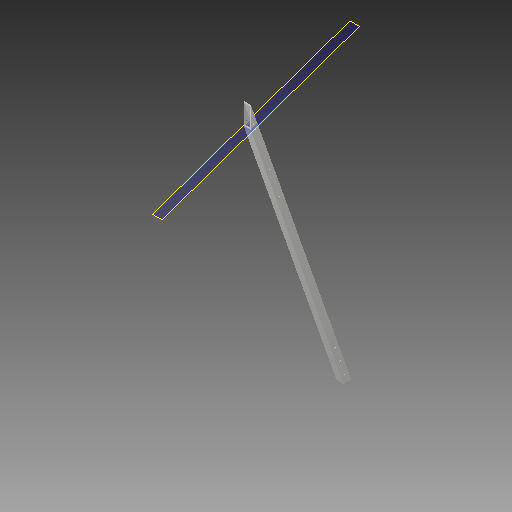
# Autodesk Inventor part: Elevator Support
Saved by Autodesk Inventor 2019.4 (Build 234330000, 330)
## iProperties
Created: 2020-01-09
Part Number: Elevator Support
Material: Aluminum 6061
Document SubType Name: Modeling
Designer: Mark
Mass: 505.998 g
Surface Area: 1886.44 cm^2
Volume: 187.407 cm^3
Density: 2.7 g/cm^3
Appearance: Aluminum - Flat
Author: Mark
Autodesk Inventor part; units mm, degrees
ref_plane "YZ Plane" through (0, 0, 0) normal (1, 0, 0) x (0, 1, 0)
ref_plane "XZ Plane" through (0, 0, 0) normal (0, 1, 0) x (-1, 0, 0)
ref_plane "XY Plane" through (0, 0, 0) normal (0, 0, 1) x (1, 0, 0)
sketch "Sketch2" plane through (0, 0, 0) normal (1, 0, 0) x (0, 1, 0)
  line L0 (0, 0) -> (75.8795, 0)
  line L1 (0, 0) -> (75.8795, 0) construction
  line L2 (-927.1205, -323.5216) -> (-927.1205, -350)
  line L3 (-927.1205, -323.5216) -> (-900.6421, -323.5216) construction
  line L4 (75.8795, 0) -> (-927.1205, -350)
  line L5 (75.8795, 0) -> (-927.1205, -350)
  line L6 (-927.1205, -323.5216) -> (0, 0)
  line L7 (0, 0) -> (75.8795, 0)
  line L8 (-927.1205, -350) -> (-927.1205, -323.5216)
  line L9 (0, 0) -> (-927.1205, -323.5216)
  line L10 (-927.1205, -350) -> (75.8795, 0)
  line L11 (75.8795, 0) -> (0, 0)
  line L12 (-927.1205, -323.5216) -> (-927.1205, -350)
  dimension "d7" = 0
  dimension "d9" = 90
  dimension "d10" = 1003
  dimension "d11" = 350
  dimension "d13" = 25
  constraints: 26 end point, 5 collinear, 4 point on line, 3 horizontal, 2 equal length, 2 parallel, 1 perpendicular, 1 vertical
  measures "d7" distance between parallel lines of L0 L1
  measures "d9" angle of L2 L3
  measures "d10" horizontal distance of L2.start L0.end
  measures "d11" vertical distance of L2.end L0.end
  measures "d13" distance between parallel lines of L4 L6
extrude "Extrusion2" add sketch "Sketch2" along normal blind 25
ref_plane "Work Plane1" through (0, 0, 0) normal (0, -0.9441661, -0.3294697) x (1, 0, 0)
sketch "Sketch3" plane through (0, 0, 0) normal (0, -0.9441661, -0.3294697) x (1, 0, 0)
  line L0 (2, -23) -> (23, -23)
  line L1 (23, -23) -> (23, -2)
  line L2 (23, -2) -> (2, -2)
  line L3 (2, -2) -> (2, -23)
  line L4 (2, -23) -> (23, -2) construction
  line L5 (23, -23) -> (2, -2) construction
  line L6 (25, -25) -> (25, 0) projected
  line L7 (0, 0) -> (25, 0) projected
  point P0 (12.5, -12.5)
  dimension "d17" = 21
  dimension "d18" = 21
  dimension "d19" = 2
  dimension "d20" = 23
  constraints: 12 end point, 2 midpoint, 2 parallel, 1 horizontal, 1 perpendicular
  measures "d17" distance of L2.end L1.end
  measures "d18" distance of L1.end L0.end
  measures "d19" distance between parallel lines of L6 L1
  measures "d20" distance between parallel lines of L7 L0
extrude "Extrusion3" cut sketch "Sketch3" along normal mid plane 2115.25
sketch "Sketch4" plane through (0, 0, 0) normal (-1, 0, 0) x (0, 0, 1)
  circle A0 centre (-65.5822, -150) radius 2.75
  circle A1 centre (-100.1765, -249.1374) radius 2.75
  line L0 (-323.5216, -927.1205) -> (0, 0) projected
  line L1 (-100.1765, -249.1374) -> (-65.5822, -150)
  dimension "d23" = 5.5
  dimension "d24" = 5.5
  dimension "d25" = 12.5
  dimension "d26" = 12.5
  dimension "d27" = 105
  dimension "d40" = 150
  constraints: 2 centre point, 2 coincident, 2 end point
  measures "d23" diameter of A0
  measures "d24" diameter of A1
  measures "d25" distance from line of L0 A1.centre
  measures "d26" distance from line of L0 A0.centre
  measures "d27" distance of L1.start L1.end
  measures "d40" vertical distance of L0.end A0.centre
extrude "Extrusion4" cut sketch "Sketch4" against normal blind 25
sketch "Sketch5" plane through (0, 0, 0) normal (-1, 0, 0) x (0, 0, 1)
  circle A0 centre (-326.2922, -897.1205) radius 2.75
  circle A1 centre (-309.8187, -849.9122) radius 2.75
  line L0 (-326.2922, -897.1205) -> (-309.8187, -849.9122)
  line L1 (-323.5216, -927.1205) -> (0, 0) projected
  line L2 (-350, -927.1205) -> (-323.5216, -927.1205) projected
  circle A2 centre (-293.3452, -802.7039) radius 2.75
  line L3 (-309.8187, -849.9122) -> (-293.3452, -802.7039)
  circle A3 centre (-15.4866, -6.4404) radius 2.75
  line L4 (0, 75.8795) -> (-350, -927.1205) projected
  line L5 (-15.4866, -6.4404) -> (-293.3452, -802.7039)
  circle A4 centre (-8.8972, 12.4429) radius 2.75
  line L6 (-15.4866, -6.4404) -> (-8.8972, 12.4429)
  dimension "d31" = 5.5
  dimension "d32" = 5.5
  dimension "d33" = 50
  dimension "d34" = 12.5
  dimension "d35" = 30
  dimension "d36" = 5.5
  dimension "d37" = 50
  dimension "d41" = 5.5
  dimension "d42" = 12.5
  dimension "d43" = 843.351
  dimension "d44" = 5.5
  dimension "d45" = 12.5
  dimension "d46" = 20
  constraints: 8 end point, 5 centre point, 4 coincident, 2 parallel
  measures "d31" diameter of A0
  measures "d32" diameter of A1
  measures "d33" distance of L0.start L0.end
  measures "d34" distance between parallel lines of L1 L0
  measures "d35" distance from line of L2 A0.centre
  measures "d36" diameter of A2
  measures "d37" distance of L0.end L3.end
  measures "d41" diameter of A3
  measures "d42" distance from line of L4 L5.start
  measures "d43" distance of L3.end L5.start
  measures "d44" diameter of A4
  measures "d45" distance from line of L4 A4.centre
  measures "d46" distance of L5.start L6.end
extrude "Extrusion5" cut sketch "Sketch5" against normal blind 25
body "Solid2"
